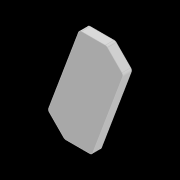
# Autodesk Inventor part: switchback-pickup-cover-8
Saved by Autodesk Inventor 2020 (Build 240168000, 168)
## iProperties
Created: 2020-01-09
Part Number: switchback-pickup-cover-8
Material: Generic
Document SubType Name: Modeling
Designer: valer
Density: 1 g/cm^3
Appearance: Default
Author: valer
Autodesk Inventor part; units mm, degrees
ref_plane "YZ Plane" through (0, 0, 0) normal (1, 0, 0) x (0, 1, 0)
ref_plane "XZ Plane" through (0, 0, 0) normal (0, 1, 0) x (-1, 0, 0)
ref_plane "XY Plane" through (0, 0, 0) normal (0, 0, 1) x (1, 0, 0)
sketch "TopProfile" plane through (0, 0, 0) normal (0, 0, 1) x (1, 0, 0)
  line L0 (22.417, 108.5547) -> (40.2604, 90.5219)
  line L1 (-6.7187, 108.5547) -> (22.417, 108.5547)
  line L2 (-6.7187, 108.5547) -> (-40.2084, 18.0328)
  line L3 (40.2604, 90.5219) -> (6.7706, 0)
  line L4 (-22.3651, 0) -> (6.7706, 0)
  line L5 (-40.2084, 18.0328) -> (-22.3651, 0)
  line L6 (-35.2804, 13.0524) -> (0.052, 108.5547) construction
  line L7 (0.052, 108.5547) -> (35.3323, 95.5023) construction
  line L8 (35.3323, 95.5023) -> (0, 0) construction
  line L9 (0, 0) -> (-35.2804, 13.0524) construction
  line L10 (-56.3022, 0) -> (56.3541, 0) construction
  line L11 (-38.1479, 18.4782) -> (-21.6231, 1.778)
  line L12 (-21.6231, 1.778) -> (5.5327, 1.778)
  line L13 (5.5327, 1.778) -> (38.1998, 90.0765)
  line L14 (38.1998, 90.0765) -> (21.6751, 106.7767)
  line L15 (21.6751, 106.7767) -> (-5.4807, 106.7767)
  line L16 (-5.4807, 106.7767) -> (-38.1479, 18.4782)
  line L17 (-29.3346, 42.3002) -> (-28.233, 45.278)
  line L18 (-28.233, 45.278) -> (-23.945, 43.6916)
  line L19 (-23.945, 43.6916) -> (-25.0467, 40.7138)
  line L20 (-25.0467, 40.7138) -> (-29.3346, 42.3002)
  line L21 (25.0986, 67.8409) -> (29.3866, 66.2545)
  line L22 (29.3866, 66.2545) -> (28.2849, 63.2768)
  line L23 (28.2849, 63.2768) -> (23.997, 64.8632)
  line L24 (23.997, 64.8632) -> (25.0986, 67.8409)
  line L25 (16.6726, 102.4057) -> (19.6504, 101.304)
  line L26 (19.6504, 101.304) -> (21.6751, 106.7767)
  line L27 (21.6751, 106.7767) -> (18.6973, 107.8784)
  line L28 (18.6973, 107.8784) -> (16.6726, 102.4057)
  line L29 (-19.5984, 7.2507) -> (-16.6207, 6.149)
  line L30 (-16.6207, 6.149) -> (-18.6454, 0.6763)
  line L31 (-18.6454, 0.6763) -> (-21.6231, 1.778)
  line L32 (-21.6231, 1.778) -> (-19.5984, 7.2507)
  point P0 (-18.2378, 1.778)
  point P1 (18.2897, 106.7767)
  dimension "d0" = 29.1357
  dimension "d2" = 69.697
  dimension "d3" = 25
  dimension "d4" = 25
  dimension "d5" = 101.8286
  dimension "d6" = 37.6174
  dimension "d7" = 25.3686
  dimension "d8" = 1.778
  dimension "d17" = 3.175
  dimension "d18" = 25.4
  dimension "d19" = 25.4
  constraints: 64 end point, 10 parallel, 8 perpendicular, 5 collinear, 4 equal length, 4 point on line, 2 horizontal, 5 other
  measures "d0" distance of L1.start L1.end
  measures "d2" angle of L10 L8
  measures "d3" angle of L9 L5
  measures "d4" angle of L7 L0
  measures "d5" distance of L6.start L7.start
  measures "d6" distance of L7.start L7.end
  measures "d7" distance of L1.end L3.start
  measures "d8" distance between parallel lines of L2 L16
  measures "d17" distance of L29.start L29.end
  measures "d18" distance from line of L21 L13.end
  measures "d19" distance from line of L11.start L20
extrude "CapFeature" add sketch "TopProfile" along normal blind 1.778 contours L0 L3 L4 L5 L2 L1 | L16 L20 L19 L18 L15 L28 L25 L26 L14 L13 L21 L24 L23 L12 L30 L29 L32 L11 | L32 L29 L30 L12 | L12 L30 L31 | L16 L18 L19 L20 | L23 L24 L21 L13 | L28 L27 L15 | L15 L26 L25 L28
extrude "WallsFeature" add sketch "TopProfile" against normal blind 7.62 contours L0 L3 L4 L5 L2 L1 | L32 L29 L30 L12 | L12 L30 L31 | L16 L18 L19 L20 | L23 L24 L21 L13 | L28 L27 L15 | L15 L26 L25 L28
fillet "SideFilletsFeature" radius 3.175 6 edges at (-22.3651, 0, -2.921) (-40.2084, 18.0328, -2.921) (6.7706, 0, -2.921) (40.2604, 90.5219, -2.921) (22.417, 108.5547, -2.921) (-6.7187, 108.5547, -2.921)
equation "\"d19\" = d18"
body "Solid1"
